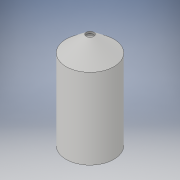
# Autodesk Inventor part: EngineMount
Saved by Autodesk Inventor 2018 (Build 220112000, 112)
## iProperties
Created: 2017-10-16
Part Number: EngineMount
Material: Generic
Document SubType Name: Modeling
Designer: Intel
Density: 1 g/cm^3
Appearance: Default
Author: Intel
Autodesk Inventor part; units mm, degrees
ref_plane "XZ Plane" through (0, 0, 0) normal (0, 1, 0) x (-1, 0, 0)
ref_plane "XY Plane" through (0, 0, 0) normal (0, 0, 1) x (1, 0, 0)
sketch "Sketch1" plane through (0, 0, 0) normal (0, 1, 0) x (-1, 0, 0)
  circle A0 centre (-12.7, -7.3323) radius 12.7
  circle A1 centre (0, 14.6647) radius 12.7
  circle A2 centre (12.7, -7.3323) radius 12.7
  circle A3 centre (0, 0) radius 36.5125
  circle A4 centre (0, 0) radius 30.1625
  line L0 (0, 14.6647) -> (-12.7, -7.3323) construction
  line L1 (-12.7, -7.3323) -> (12.7, -7.3323) construction
  line L2 (12.7, -7.3323) -> (0, 14.6647) construction
  line L3 (0, -7.3323) -> (0, 14.6647) construction
  line L4 (6.35, 3.6662) -> (-12.7, -7.3323) construction
  line L5 (-6.35, 3.6662) -> (12.7, -7.3323) construction
  line L6 (0, -7.3323) -> (0, 27.3647) construction
  circle A5 centre (0, 0) radius 27.3647 construction
  line L7 (0, -51.1175) -> (0, 51.1175) projected
  point P0 (-6.35, 3.6662)
  dimension "d0" = 25.4
  dimension "d1" = 25.4
  dimension "d2" = 25.4
  dimension "d7" = 73.025
  dimension "d8" = 6.35
  constraints: 14 end point, 5 centre point, 4 midpoint, 3 coincident, 3 equal radius, 3 point on line, 2 point on circle, 1 collinear, 1 vertical alignment, 2 other
  measures "d0" diameter of A0
  measures "d1" diameter of A1
  measures "d2" diameter of A2
  measures "d7" diameter of A3
  measures "d8" radial gap between concentric circles of A3 A4
extrude "Extrusion1" add sketch "Sketch1" along normal blind 96.52 contours L7 A4 A1 A0 | L7 A1 A2 | A2 A1 L7 A4 | A0 A1 L7
sketch "Sketch2" plane through (0, 96.52, 0) normal (0, 1, 0) x (1, 0, 0)
  circle A0 centre (0, 0) radius 30.1625
  constraints: 1 centre point, 1 coincident
ref_plane "Work Plane2" through (0, 0, 0) normal (1, 0, 0) x (0, 1, 0)
sketch "Sketch4" plane through (0, 0, 0) normal (1, 0, 0) x (0, 1, 0)
  line L0 (96.52, -30.1625) -> (96.52, 30.1625) projected
  line L1 (96.52, 4.7625) -> (121.92, 4.7625)
  line L2 (96.52, -30.1625) -> (96.52, 30.1625) projected
  line L3 (0, 30.1625) -> (0, -30.1625) projected
  line L4 (96.52, -30.1625) -> (96.52, 30.1625) projected
  line L5 (0, 30.1625) -> (0, -30.1625) projected
  line L6 (0, 30.1625) -> (96.52, 30.1625) projected
  line L7 (96.52, 4.7625) -> (96.52, 30.1625)
  line L8 (96.52, 30.1625) -> (101.6, 30.1625)
  line L9 (101.6, 30.1625) -> (121.92, 4.7625)
  line L10 (96.52, 0) -> (123.5586, 0)
  line L11 (101.092, 27.6225) -> (119.38, 4.7625)
  line L12 (96.52, 27.6225) -> (101.092, 27.6225)
  line L13 (96.52, 27.6225) -> (96.52, 30.1625)
  point P0 (0, 0)
  dimension "d14" = 25.4
  dimension "d15" = 25.4
  dimension "d16" = 5.08
  dimension "d18" = 4.7625
  dimension "d19" = 2.54
  constraints: 16 end point, 3 horizontal, 3 point on line, 2 collinear, 1 midpoint, 1 parallel, 1 perpendicular
  measures "d14" distance of L1.start L1.end
  measures "d15" distance between parallel lines of L6 L1
  measures "d16" distance of L6.end L8.end
  measures "d18" distance between parallel lines of L10 L1
  measures "d19" distance between parallel lines of L8 L12
revolve "Revolution1" add sketch "Sketch4" angle 360 about axis through (0, 96.52, 0) along (0, 1, 0) contours L0 L8 L9 L1 L11 L12
equation "\"d0\" = d1"
equation "\"d2\" = d1"
body "Solid1"
